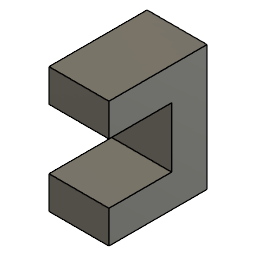
replay (Autodesk Fusion 360 design; units mm, degrees)
Autodesk Fusion 360 part; units mm, degrees
ref_plane "工作平面1" through (25, 0, 0) normal (1, 0, 0) x (0, 1, 0)
sketch "草图1" plane through (25, 0, 0) normal (1, 0, 0) x (0, 0, -1)
  line L0 (-36, 12) -> (-13, 12)
  line L1 (-13, 12) -> (-13, 34)
  line L2 (-13, 34) -> (-36, 34)
  line L3 (-36, 34) -> (-36, 46)
  line L4 (-36, 46) -> (0, 46)
  line L5 (0, 46) -> (0, 0)
  line L6 (0, 0) -> (-36, 0)
  line L7 (-36, 0) -> (-36, 12)
extrude "拉伸1" add sketch "草图1" against normal blind 22
